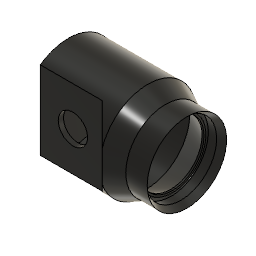
3-012 Cap for Gland (Autodesk Fusion 360 design; units mm, degrees)
Autodesk Fusion 360 part; units mm, degrees
note: some values were not read from the file. Set by a fixed rule: which sketch regions a step uses.
sketch "Sketch1" plane through (0, 0, 0) normal (0, 1, 0) x (1, 0, 0)
  line L0 (-228.9333, 20.65) -> (-224.0621, 18.3051)
  arc A0 (-224.0621, 18.3051) -> (-223.0369, 18.3695) centre (-223.6869, 20.5235) ccw
  line L1 (-223.0369, 18.3695) -> (-223.0369, 19.4735)
  line L2 (-223.0369, 19.4735) -> (-223.6869, 19.4735)
  arc A1 (-223.6869, 19.4735) -> (-223.7427, 21.5721) centre (-223.6869, 20.5235) cw
  line L3 (-223.7427, 21.5721) -> (-218.5269, 21.85)
  line L4 (-218.5269, 21.85) -> (-217.9673, 20.65)
  line L5 (-217.9673, 20.65) -> (-214.5397, 23.05)
  line L6 (-214.5397, 23.05) -> (-242.49, 23.05)
  line L7 (-242.49, 23.05) -> (-249.49, 16.05)
  line L8 (-246.99, 14.3074) -> (-240.6474, 20.65)
  line L9 (-240.6474, 20.65) -> (-228.9333, 20.65)
  line L10 (-224.0621, -18.3051) -> (-228.9333, -20.65)
  line L11 (-242.49, -23.05) -> (-214.5397, -23.05)
  line L12 (-214.5397, -23.05) -> (-217.9673, -20.65)
  line L13 (-217.9673, -20.65) -> (-218.5269, -21.85)
  line L14 (-218.5269, -21.85) -> (-223.7427, -21.5721)
  arc A2 (-223.7427, -21.5721) -> (-223.6869, -19.4735) centre (-223.6869, -20.5235) cw
  line L15 (-223.6869, -19.4735) -> (-223.0369, -19.4735)
  line L16 (-223.0369, -19.4735) -> (-223.0369, -18.3695)
  arc A3 (-223.0369, -18.3695) -> (-224.0621, -18.3051) centre (-223.6869, -20.5235) ccw
  line L17 (0, 0) -> (-313.6932, 0)
  line L18 (-228.9333, -20.65) -> (-237.9696, -25)
  line L19 (-237.9696, -25) -> (-280.5397, -25)
  line L20 (-227.0024, -23.05) -> (-237.2851, -28)
  line L21 (-237.2851, -28) -> (-283.5397, -28)
  circle A4 centre (-264.5397, 0) radius 8.5
  circle A5 centre (-264.5397, 0) radius 16
  circle A6 centre (-264.5397, 0) radius 19
  line L22 (-283.5397, 0) -> (-283.5397, -28)
  line L23 (-280.5397, 0) -> (-280.5397, -25)
  dimension "d228" = 3
  dimension "d229" = 3
  dimension "d231" = 25
  dimension "d232" = 17
  dimension "d233" = 32
  dimension "d234" = 50
  dimension "d235" = 3
  constraint coincident L17.start origin
  constraint horizontal L17
  constraint coincident L10.end L18.start
  constraint parallel L10 L18
  constraint parallel L11 L19
  constraint coincident L11 L20.start
  constraint parallel L11 L21
  constraint parallel L18 L20
  constraint coincident L17 A4.centre
  constraint concentric A4 A5
  constraint concentric A5 A6
  constraint coincident A6 L22.start
  constraint tangent A6 L22
  constraint coincident A5 L23.start
  constraint tangent A5 L23
  constraint parallel L22 L23
  constraint vertical L22
  measures "d228" distance of L18 L20
  measures "d229" distance of L19 L21
  measures "d231" distance of L17 L19
  measures "d232" diameter of A4
  measures "d233" diameter of A5
  measures "d234" horizontal distance of L11.end A4.centre
  measures "d235" distance of A5 A6
revolve "Revolve1" add sketch "Sketch1" angle 360 about axis through (0, 0, 0) along (-1, 0, 0) contours L10 L11 L12 L13 L14 A2 L15 L16 A3 L18 | L11 L18 L19 L20 L21 A6 L22 L23 | L17 A6 L23
extrude "Extrude1" cut sketch "Sketch1" against normal blind 35 contours L17 A4 | L17 A4
sketch "Sketch2" plane through (-283.5397, 0, 0) normal (-1, 0, 0) x (0, -1, 0)
  circle A0 centre (0, 0) radius 28
  line L0 (0, 19) -> (0, -19)
  circle A1 centre (0, 0) radius 25
  line L1 (0, 19) -> (16.2481, 19)
  line L2 (0, -19) -> (16.2481, -19)
  line L3 (16.2481, 22.8035) -> (16.2481, -22.8035)
  line L4 (13.2481, 24.6676) -> (13.2481, -24.6676)
  dimension "d240" = 3
  constraint coincident L0.start L1.start
  constraint coincident A1 L1.end
  constraint perpendicular L0 L1
  constraint coincident L0.end L2.start
  constraint coincident A1 L2.end
  constraint perpendicular L0 L2
  constraint coincident A0 L3.start
  constraint coincident A0 L3.end
  constraint vertical L3
  constraint coincident L2.end L3
  constraint coincident A0 L4.start
  constraint coincident A0 L4.end
  constraint perpendicular L2 L4
  measures "d240" distance of L3 L4
ref_plane "WorkPlane1" through (0, -16.2481, 0) normal (0, 1, 0) x (0, 0, 1)
extrude "Extrude2" add sketch "Sketch2" against normal blind 39 contours A0 A1 L3 | A0 A1 L3 L4 | A0 A1 L3 L4 | A1 L1 L4 | L1 L2 L3 L4 | A1 L3 | A1 L2 L4
extrude "Extrude3" cut sketch "Sketch2" against normal up to surface (36 mm away) contours A0 A1 L3 | A1 L3
extrude "Extrude4" cut sketch "Sketch1" against normal blind 46 contours L17 A4 | L17 A4
extrude "Extrude5" add 1 faces at (-244.5397, -17.1654, 0) along direction (1, 0, 0) blind 8
sketch "Sketch3" plane through (0, 0, 0) normal (0, 0, 1) x (1, 0, 0)
  line L0 (-256.0397, -13.2481) -> (-256.0397, -16.2481)
  line L1 (-256.0397, -16.2481) -> (-247.5397, -16.2481)
  line L2 (-247.5397, -16.2481) -> (-247.5397, -28)
  line L3 (-247.5397, -28) -> (-237.2851, -28)
  line L4 (-237.2851, -28) -> (-227.0024, -23.05)
  line L5 (-227.0024, -23.05) -> (-214.5397, -23.05)
  line L6 (-214.5397, -23.05) -> (-217.9673, -20.65)
  line L7 (-217.9673, -20.65) -> (-218.5269, -21.85)
  line L8 (-218.5269, -21.85) -> (-223.7427, -21.5721)
  arc A0 (-223.7427, -21.5721) -> (-223.6869, -19.4735) centre (-223.6869, -20.5235) cw
  line L9 (-223.6869, -19.4735) -> (-223.0369, -19.4735)
  line L10 (-223.0369, -19.4735) -> (-223.0369, -18.3695)
  arc A1 (-223.0369, -18.3695) -> (-224.0621, -18.3051) centre (-223.6869, -20.5235) ccw
  line L11 (-224.0621, -18.3051) -> (-236.5397, -24.3117)
  line L12 (-236.5397, -24.3117) -> (-236.5397, -13.2481)
  line L13 (-236.5397, -13.2481) -> (-256.0397, -13.2481)
  line L14 (-237.2851, 28) -> (-283.5397, 28)
  line L15 (-283.5397, 28) -> (-283.5397, -16.2481)
  line L16 (-283.5397, -16.2481) -> (-273.0397, -16.2481)
  line L17 (-273.0397, -16.2481) -> (-273.0397, -13.2481)
  line L18 (-273.0397, -13.2481) -> (-280.5397, -13.2481)
  line L19 (-280.5397, -13.2481) -> (-280.5397, 25)
  line L20 (-237.9696, 25) -> (-224.0621, 18.3051)
  arc A2 (-224.0621, 18.3051) -> (-223.0369, 18.3695) centre (-223.6869, 20.5235) ccw
  line L21 (-223.0369, 18.3695) -> (-223.0369, 19.4735)
  line L22 (-223.0369, 19.4735) -> (-223.6869, 19.4735)
  arc A3 (-223.6869, 19.4735) -> (-223.7427, 21.5721) centre (-223.6869, 20.5235) cw
  line L23 (-223.7427, 21.5721) -> (-218.5269, 21.85)
  line L24 (-218.5269, 21.85) -> (-217.9673, 20.65)
  line L25 (-217.9673, 20.65) -> (-214.5397, 23.05)
  line L26 (-214.5397, 23.05) -> (-227.0024, 23.05)
  line L27 (-227.0024, 23.05) -> (-237.2851, 28)
  line L28 (-247.5397, -16.2481) -> (-235.7878, -28)
  line L29 (-280.5397, 25) -> (-237.9696, 25)
  dimension "d252" = 45
  constraint coincident L1.end L2.start
  constraint coincident L3 L28.end
  measures "d252" angle of L2 L28
extrude "Extrude6" cut sketch "Sketch3" along normal mid plane 80 contours L2 L3 L4 L28
chamfer "Chamfer2" distance 3 angle 45 1 edges at (-236.5397, -24.3117, 0)
